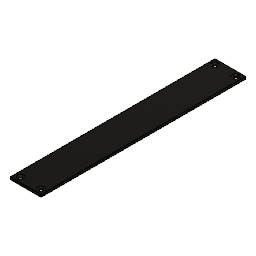
LED Light Holder Assembly (Autodesk Fusion 360 archive; units mm, degrees)
design "LED Light Holder Middle"
Autodesk Fusion 360 part; units mm, degrees
box "BoxPrimitive1" add length 200 width 30 height 5 placed x (0, 0, -1) y (-1, 0, 0) z (0, 1, 0) at (20, 0, 130) in component "Component"
sketch "Sketch2" plane through (0, 5, 0) normal (0, 1, 0) x (-1, 0, 0) in component "Component"
  line L0 (-20, -70) -> (10, -70)
  line L1 (10, -70) -> (10, 130)
  line L2 (10, 130) -> (-20, 130)
  line L3 (-20, 130) -> (-20, -70)
  point P0 (-15, -65)
  point P1 (5, -65)
  point P2 (-15, 125)
  point P3 (5, 125)
  dimension "d19" = 20
  dimension "d20" = 5
  dimension "d21" = 5
  dimension "d22" = 5
  constraint horizontal P2 P3
  constraint horizontal P0 P1
  constraint vertical P1 P3
  constraint vertical P0 P2
  measures "d19" distance of P2 P3
  measures "d20" distance of L3 P2
  measures "d21" distance of L2 P2
  measures "d22" distance of L0 P0
hole "Hole1" at (15, 5, -65) at (-5, 5, -65) at (-5, 5, 125) at (15, 5, 125) direction (0, -1, 0) diameter 3.4 depth 12 tip angle 118 countersink diameter 6.3 countersink angle 90 in component "Component"
extrude "Extrude1" cut 1 faces at (8.2675, 0, -1.0962) along direction (0, 1, 0) blind 2.5 in component "Component"
extrude "Extrude2" cut 1 faces at (8.2675, 2.5, -1.0962) along direction (0, 1, 0) blind 0.1 in component "Component"
component "Component" placed x (1, 0, 0) y (0, 1, 0) z (0, 0, 1) at (0, 0, 0)

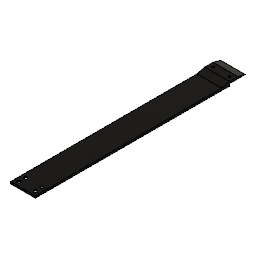
design "LED Light Holder Side"
Autodesk Fusion 360 part; units mm, degrees
form "Form1" [no effect] in component "Component"
box "BoxPrimitive1" add length 250 width 30 height -20 placed x (0, 0, -1) y (-1, 0, 0) z (0, 1, 0) at (30, 0, -100) in component "Component"
move_face "OffsetFaces1" offset -15 1 faces at (10, 0, -183.3333) in component "Component"
sketch "Sketch9" plane through (0, -20, 0) normal (0, -1, 0) x (1, 0, 0) in component "Component"
  line L0 (30, -100) -> (0, -100)
  line L1 (0, -100) -> (0, -350)
  line L2 (0, -350) -> (30, -350)
  line L3 (30, -350) -> (30, -100)
  point P0 (5, -120)
  point P1 (25, -120)
  point P2 (5, -128)
  point P3 (25, -128)
  dimension "d31" = 20
  dimension "d32" = 5
  dimension "d33" = 8
  dimension "d49" = 20
  constraint horizontal P0 P1
  constraint vertical P0 P2
  constraint horizontal P2 P3
  constraint vertical P1 P3
  measures "d31" distance of P0 P1
  measures "d32" distance of L1 P2
  measures "d33" distance of P0 P2
  measures "d49" distance of L0 P1
hole "Hole4" at (25, -20, -120) at (5, -20, -120) at (5, -20, -128) at (25, -20, -128) direction (0, 1, 0) diameter 3.797 depth 9 tip angle 180 countersink diameter 7.087 countersink angle 82 in component "Component"
extrude "Extrude4" cut 1 faces at (20, -18.3333, -350) along direction (0, 0, 1) blind 0.05 in component "Component"
extrude "Extrude5" cut 1 faces at (11.6667, -15, -276.5995) along direction (0, -1, 0) blind 2.5 in component "Component"
sketch "Sketch10" plane through (30, 0, 0) normal (1, 0, 0) x (0, 0, -1) in component "Component"
  line L0 (349.95, -17.5) -> (100, -17.5)
  line L1 (100, -17.5) -> (100, -20)
  line L2 (100, -20) -> (349.95, -20)
  line L3 (349.95, -20) -> (349.95, -17.5)
  line L4 (349.95, -17.5) -> (362.45, -17.5)
  line L5 (362.45, -17.5) -> (362.45, -15)
  line L6 (362.45, -15) -> (349.95, -15)
  line L7 (349.95, -15) -> (349.95, -17.5)
  line L8 (349.95, -15) -> (340.6199, -17.5)
  line L9 (362.45, -17.5) -> (372.45, -17.5)
  line L10 (359.95, -15) -> (369.2801, -17.5)
  dimension "d38" = 2.5
  dimension "d39" = 12.5
  dimension "d41" = 75
  dimension "d52" = 10
  dimension "d54" = 15
  dimension "d55" = 10
  constraint horizontal L4
  constraint vertical L5
  constraint horizontal L6
  constraint vertical L7
  constraint coincident L0 L3.end
  constraint vertical L2.end L6.end
  constraint coincident L0 L8.end
  constraint perpendicular L5 L9
  constraint coincident L6 L10.start
  constraint coincident L9 L10.end
  measures "d38" distance of L4 L6
  measures "d39" distance of L5 L7
  measures "d41" angle of L7 L8
  measures "d52" distance of L4.end L9.end
  measures "d54" angle of L6 L10
  measures "d55" distance of L6.end L10.start
extrude "Extrude6" add sketch "Sketch10" against normal blind 30 contours L4 L5 L6 L7 L10 | L0 L7 L8 | L5 L9 L10 in component "Component"
sketch "Sketch11" plane through (0, -15, 0) normal (0, 1, 0) x (-1, 0, 0) in component "Component"
  line L0 (-30, -349.95) -> (-30, -359.95)
  line L1 (0, -359.95) -> (0, -349.95)
  line L2 (0, -349.95) -> (-30, -349.95)
  line L3 (0, -349.95) -> (-30, -349.95)
  line L4 (-30, -359.95) -> (0, -359.95)
  point P0 (-5, -355)
  point P1 (-25, -355)
  dimension "d44" = 20
  dimension "d45" = 5
  dimension "d46" = 5.05
  constraint horizontal P0 P1
  measures "d44" distance of P0 P1
  measures "d45" distance of L0 P1
  measures "d46" distance of P1 L3
hole "Hole5" at (25, -15, -355) at (5, -15, -355) direction (0, -1, 0) diameter 2.85 end through all in component "Component"
extrude "Extrude7" cut 1 faces at (20, -19.1667, -100) along direction (0, 0, -1) blind 15 in component "Component"
component "Component" placed x (1, 0, 0) y (0, 1, 0) z (0, 0, 1) at (0, 0, 0)
